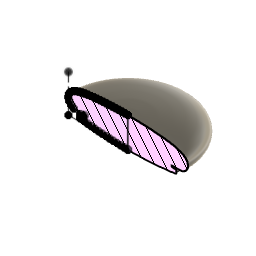
AirTag (Autodesk Fusion 360 design; units mm, degrees)
Autodesk Fusion 360 part; units mm, degrees
sketch "AirTag profile" plane through (0, 0, 0) normal (0, 1, 0) x (1, 0, 0)
  line L0 (-15.93, -10) -> (-15.93, 0) construction
  line L1 (0, 0) -> (-15.93, 0) construction
  line L2 (0, 0) -> (0, -7.98)
  line L3 (-12.72, -0.88) -> (-12.77, -0.93)
  line L4 (-12.77, -0.93) -> (-12.77, -1.84)
  line L5 (-12.77, -1.84) -> (-12.72, -1.89)
  line L6 (-12.72, -1.89) -> (-11.555, -1.89)
  line L7 (-11.555, -1.89) -> (-11.555, -2.29)
  line L8 (-11.555, -2.29) -> (-14.47, -2.29)
  spline S0 degree 5 poles (0, 0) (-0.0393, -0.0007) (-0.118, -0.002) (-0.2358, -0.0038) (-0.3929, -0.0059) (-0.589, -0.0078) (-0.7849, -0.0091) (-0.9807, -0.01) (-1.1764, -0.0108) (-1.3722, -0.0118) (-1.5682, -0.0134) (-1.7645, -0.0159) (-1.9612, -0.0197) (-2.1583, -0.0247) (-2.3557, -0.0307) (-2.5531, -0.0372) (-2.7505, -0.0438) (-2.9476, -0.05) (-3.1443, -0.0558) (-3.3406, -0.0612) (-3.5366, -0.0666) (-3.7323, -0.0726) (-3.928, -0.0796) (-4.1237, -0.0878) (-4.3195, -0.0972) (-4.5155, -0.1076) (-4.7117, -0.1186) (-4.9081, -0.1299) (-5.1045, -0.1412) (-5.3009, -0.1527) (-5.4971, -0.1645) (-5.6928, -0.1768) (-5.8881, -0.1897) (-6.083, -0.2033) (-6.2776, -0.2175) (-6.4721, -0.2319) (-6.6668, -0.2462) (-6.8618, -0.2602) (-7.0572, -0.2738) (-7.2531, -0.2872) (-7.4492, -0.3007) (-7.6454, -0.3148) (-7.8415, -0.3298) (-8.0375, -0.346) (-8.2332, -0.3634) (-8.4289, -0.3817) (-8.6245, -0.4006) (-8.8204, -0.42) (-9.0164, -0.4395) (-9.2124, -0.4592) (-9.4083, -0.4791) (-9.6039, -0.4992) (-9.799, -0.5198) (-9.9937, -0.5408) (-10.188, -0.5624) (-10.3822, -0.5846) (-10.5765, -0.6071) (-10.7711, -0.6301) (-10.9661, -0.6533) (-11.1616, -0.6769) (-11.3573, -0.7008) (-11.5532, -0.7251) (-11.7489, -0.7497) (-11.9442, -0.7748) (-12.139, -0.8004) (-12.3333, -0.8264) (-12.4883, -0.8476) (-12.6043, -0.8637) (-12.6814, -0.8746) (-12.72, -0.88) knots 0 0 0 0 0 0 0.01538462 0.03076923 0.04615385 0.06153846 0.07692308 0.09230769 0.10769231 0.12307692 0.13846154 0.15384615 0.16923077 0.18461538 0.2 0.21538462 0.23076923 0.24615385 0.26153846 0.27692308 0.29230769 0.30769231 0.32307692 0.33846154 0.35384615 0.36923077 0.38461538 0.4 0.41538462 0.43076923 0.44615385 0.46153846 0.47692308 0.49230769 0.50769231 0.52307692 0.53846154 0.55384615 0.56923077 0.58461538 0.6 0.61538462 0.63076923 0.64615385 0.66153846 0.67692308 0.69230769 0.70769231 0.72307692 0.73846154 0.75384615 0.76923077 0.78461538 0.8 0.81538462 0.83076923 0.84615385 0.86153846 0.87692308 0.89230769 0.90769231 0.92307692 0.93846154 0.95384615 0.96923077 0.98461538 1 1 1 1 1 1
  spline S1 degree 5 poles (-14.47, -2.29) (-14.4999, -2.3052) (-14.5592, -2.3362) (-14.6468, -2.3846) (-14.7609, -2.4529) (-14.8991, -2.5447) (-15.0325, -2.643) (-15.1609, -2.7478) (-15.2835, -2.8595) (-15.3993, -2.9782) (-15.5072, -3.1043) (-15.6057, -3.238) (-15.6936, -3.3793) (-15.7695, -3.5277) (-15.8323, -3.6825) (-15.8811, -3.8424) (-15.9152, -4.0061) (-15.934, -4.172) (-15.9374, -4.3386) (-15.9254, -4.5046) (-15.8984, -4.6687) (-15.8567, -4.8296) (-15.8012, -4.9864) (-15.7327, -5.138) (-15.6519, -5.2835) (-15.56, -5.4222) (-15.458, -5.5536) (-15.347, -5.6772) (-15.2281, -5.793) (-15.1023, -5.9012) (-14.9707, -6.0023) (-14.8344, -6.0968) (-14.6941, -6.1854) (-14.5505, -6.2687) (-14.4043, -6.3469) (-14.2558, -6.4204) (-14.1053, -6.4894) (-13.953, -6.5541) (-13.7991, -6.6147) (-13.6439, -6.6715) (-13.4874, -6.7249) (-13.3299, -6.7754) (-13.1715, -6.8231) (-13.0124, -6.8686) (-12.8527, -6.9121) (-12.6925, -6.9538) (-12.5319, -6.9939) (-12.3711, -7.0325) (-12.2099, -7.0696) (-12.0483, -7.1053) (-11.8864, -7.1393) (-11.7239, -7.1716) (-11.561, -7.2021) (-11.3975, -7.2308) (-11.2337, -7.2579) (-11.0698, -7.2835) (-10.9058, -7.3079) (-10.7419, -7.3313) (-10.5782, -7.354) (-10.4145, -7.3762) (-10.2507, -7.3981) (-10.0865, -7.4197) (-9.9219, -7.4411) (-9.7567, -7.4623) (-9.5913, -7.483) (-9.4257, -7.5031) (-9.2603, -7.5224) (-9.0954, -7.5407) (-8.9309, -7.5581) (-8.7668, -7.5745) (-8.6028, -7.5903) (-8.4386, -7.6056) (-8.2739, -7.6206) (-8.1087, -7.6354) (-7.9431, -7.6499) (-7.7772, -7.664) (-7.6115, -7.6776) (-7.446, -7.6905) (-7.2811, -7.7027) (-7.1166, -7.7145) (-6.9524, -7.7262) (-6.7882, -7.7381) (-6.6238, -7.7504) (-6.459, -7.7631) (-6.2937, -7.7759) (-6.128, -7.7884) (-5.9619, -7.8001) (-5.7957, -7.8106) (-5.6295, -7.8198) (-5.4634, -7.8278) (-5.2976, -7.8353) (-5.1321, -7.8425) (-4.9671, -7.85) (-4.8025, -7.858) (-4.638, -7.8664) (-4.4737, -7.8749) (-4.3091, -7.883) (-4.1443, -7.8905) (-3.979, -7.897) (-3.8134, -7.903) (-3.6475, -7.9085) (-3.4815, -7.9141) (-3.3154, -7.9201) (-3.1495, -7.9265) (-2.9837, -7.9332) (-2.818, -7.9397) (-2.6524, -7.9456) (-2.4868, -7.9504) (-2.3211, -7.954) (-2.1553, -7.9563) (-1.9895, -7.9579) (-1.8237, -7.9589) (-1.6578, -7.9599) (-1.492, -7.9613) (-1.3262, -7.963) (-1.1604, -7.9651) (-0.9947, -7.9675) (-0.8289, -7.97) (-0.6632, -7.9725) (-0.4974, -7.9748) (-0.3316, -7.9768) (-0.199, -7.9782) (-0.0995, -7.9792) (-0.0332, -7.9797) (0, -7.98) knots 0 0 0 0 0 0 0.00833333 0.01666667 0.025 0.03333333 0.04166667 0.05 0.05833333 0.06666667 0.075 0.08333333 0.09166667 0.1 0.10833333 0.11666667 0.125 0.13333333 0.14166667 0.15 0.15833333 0.16666667 0.175 0.18333333 0.19166667 0.2 0.20833333 0.21666667 0.225 0.23333333 0.24166667 0.25 0.25833333 0.26666667 0.275 0.28333333 0.29166667 0.3 0.30833333 0.31666667 0.325 0.33333333 0.34166667 0.35 0.35833333 0.36666667 0.375 0.38333333 0.39166667 0.4 0.40833333 0.41666667 0.425 0.43333333 0.44166667 0.45 0.45833333 0.46666667 0.475 0.48333333 0.49166667 0.5 0.50833333 0.51666667 0.525 0.53333333 0.54166667 0.55 0.55833333 0.56666667 0.575 0.58333333 0.59166667 0.6 0.60833333 0.61666667 0.625 0.63333333 0.64166667 0.65 0.65833333 0.66666667 0.675 0.68333333 0.69166667 0.7 0.70833333 0.71666667 0.725 0.73333333 0.74166667 0.75 0.75833333 0.76666667 0.775 0.78333333 0.79166667 0.8 0.80833333 0.81666667 0.825 0.83333333 0.84166667 0.85 0.85833333 0.86666667 0.875 0.88333333 0.89166667 0.9 0.90833333 0.91666667 0.925 0.93333333 0.94166667 0.95 0.95833333 0.96666667 0.975 0.98333333 0.99166667 1 1 1 1 1 1
  point P0 (-15.93, 0)
  point P1 (0, -7.98)
  point P2 (-0.83, -7.97)
  point P3 (-1.66, -7.96)
  point P4 (-3.32, -7.92)
  point P5 (-2.49, -7.95)
  point P6 (-4.15, -7.89)
  point P7 (-7.45, -7.69)
  point P8 (-6.63, -7.75)
  point P9 (-4.97, -7.85)
  point P10 (-5.8, -7.81)
  point P11 (-8.28, -7.62)
  point P12 (-9.1, -7.54)
  point P13 (-9.93, -7.44)
  point P14 (-10.75, -7.33)
  point P15 (-11.57, -7.2)
  point P16 (-12.38, -7.03)
  point P17 (-13.96, -6.55)
  point P18 (-14.7, -6.18)
  point P19 (-15.8, -4.98)
  point P20 (-15.93, -4.17)
  point P21 (-12.72, -0.88)
  point P22 (-13.18, -6.82)
  point P23 (-15.35, -5.67)
  point P24 (-14.47, -2.29)
  point P25 (-15.16, -2.75)
  point P26 (-15.69, -3.38)
  point P27 (-11.75, -0.75)
  point P28 (-10.77, -0.63)
  point P29 (-9.8, -0.52)
  point P30 (-8.82, -0.42)
  point P31 (-7.84, -0.33)
  point P32 (-6.86, -0.26)
  point P33 (-5.89, -0.19)
  point P34 (-4.91, -0.13)
  point P35 (-3.93, -0.08)
  point P36 (-2.95, -0.05)
  point P37 (-0.98, -0.01)
  point P38 (-1.96, -0.02)
  point P39 (-11.555, -2.29)
  point P40 (-11.555, -1.89)
  point P41 (-12.77, -1.84)
  point P42 (-12.72, -1.89)
  point P43 (-12.77, -0.93)
  point P44 (-0.98, -0.01)
  point P45 (-1.96, -0.02)
  point P46 (-2.95, -0.05)
  point P47 (-3.93, -0.08)
  point P48 (-4.91, -0.13)
  point P49 (-5.89, -0.19)
  point P50 (-6.86, -0.26)
  point P51 (-7.84, -0.33)
  point P52 (-8.82, -0.42)
  point P53 (-9.8, -0.52)
  point P54 (-10.77, -0.63)
  point P55 (-11.75, -0.75)
  point P56 (-15.16, -2.75)
  point P57 (-15.69, -3.38)
  point P58 (-15.93, -4.17)
  point P59 (-15.8, -4.98)
  point P60 (-15.35, -5.67)
  point P61 (-14.7, -6.18)
  point P62 (-13.96, -6.55)
  point P63 (-13.18, -6.82)
  point P64 (-12.38, -7.03)
  point P65 (-11.57, -7.2)
  point P66 (-10.75, -7.33)
  point P67 (-9.93, -7.44)
  point P68 (-9.1, -7.54)
  point P69 (-8.28, -7.62)
  point P70 (-7.45, -7.69)
  point P71 (-6.63, -7.75)
  point P72 (-5.8, -7.81)
  point P73 (-4.97, -7.85)
  point P74 (-4.15, -7.89)
  point P75 (-3.32, -7.92)
  point P76 (-2.49, -7.95)
  point P77 (-1.66, -7.96)
  point P78 (-0.83, -7.97)
  dimension "d1" = 10
  dimension "d2" = 15.93
  dimension "d3" = 15.93
  dimension "d4" = 15.1
  dimension "d5" = 14.27
  dimension "d6" = 13.44
  dimension "d7" = 12.61
  dimension "d8" = 11.78
  dimension "d9" = 10.96
  dimension "d10" = 10.13
  dimension "d11" = 9.3
  dimension "d12" = 8.48
  dimension "d13" = 7.65
  dimension "d14" = 6.83
  dimension "d15" = 6
  dimension "d16" = 5.18
  dimension "d17" = 4.36
  dimension "d18" = 3.55
  dimension "d19" = 2.75
  dimension "d20" = 1.97
  dimension "d21" = 1.23
  dimension "d22" = 0.58
  dimension "d23" = 0.13
  dimension "d24" = 7.98
  dimension "d25" = 7.97
  dimension "d26" = 7.96
  dimension "d27" = 7.95
  dimension "d28" = 7.92
  dimension "d29" = 7.89
  dimension "d30" = 7.85
  dimension "d31" = 7.81
  dimension "d32" = 7.75
  dimension "d33" = 7.69
  dimension "d34" = 7.62
  dimension "d35" = 7.54
  dimension "d36" = 7.44
  dimension "d37" = 7.33
  dimension "d38" = 7.2
  dimension "d39" = 7.03
  dimension "d40" = 6.82
  dimension "d41" = 6.55
  dimension "d42" = 6.18
  dimension "d43" = 5.67
  dimension "d44" = 4.98
  dimension "d45" = 4.17
  dimension "d46" = 0.24
  dimension "d47" = 0.77
  dimension "d48" = 1.46
  dimension "d49" = 3.21
  dimension "d50" = 4.18
  dimension "d51" = 5.16
  dimension "d52" = 6.13
  dimension "d53" = 7.11
  dimension "d54" = 8.09
  dimension "d55" = 9.07
  dimension "d56" = 10.04
  dimension "d57" = 11.02
  dimension "d58" = 12
  dimension "d59" = 12.98
  dimension "d60" = 13.97
  dimension "d61" = 14.95
  dimension "d62" = 15.93
  dimension "d63" = 0.01
  dimension "d64" = 0.02
  dimension "d65" = 0.05
  dimension "d66" = 0.08
  dimension "d67" = 0.13
  dimension "d68" = 0.19
  dimension "d69" = 0.26
  dimension "d70" = 0.33
  dimension "d71" = 0.42
  dimension "d72" = 0.52
  dimension "d73" = 0.63
  dimension "d74" = 0.75
  dimension "d75" = 0.88
  dimension "d76" = 2.29
  dimension "d77" = 2.75
  dimension "d78" = 3.38
  dimension "d79" = 11.555
  dimension "d80" = 2.29
  dimension "d81" = 1.89
  dimension "d82" = 0.05
  dimension "d83" = 0.05
  dimension "d84" = 0.05
  constraint vertical L0
  constraint horizontal L1.start L0.end
  constraint coincident L1.start L2.start
  constraint coincident P0 L0.end
  constraint coincident L0 P58
  constraint coincident P1 L2.end
  constraint vertical P39 P40
  constraint vertical P21 P42
  constraint horizontal P40 P42
  constraint vertical P41 P43
  constraint coincident P21 L3.start
  constraint coincident P43 L3.end
  constraint coincident P41 L4.end
  constraint coincident P42 L5.end
  constraint coincident P40 L6.end
  constraint coincident P39 L7.end
  constraint coincident P24 L8.end
  constraint coincident P44 P37
  constraint coincident P45 P38
  constraint coincident P46 P36
  constraint coincident P47 P35
  constraint coincident P48 P34
  constraint coincident P49 P33
  constraint coincident P50 P32
  constraint coincident P51 P31
  constraint coincident P52 P30
  constraint coincident P53 P29
  constraint coincident P54 P28
  constraint coincident P55 P27
  constraint coincident P56 P25
  constraint coincident P57 P26
  constraint coincident P58 P20
  constraint coincident P59 P19
  constraint coincident P60 P23
  constraint coincident P61 P18
  constraint coincident P62 P17
  constraint coincident P63 P22
  constraint coincident P64 P16
  constraint coincident P65 P15
  constraint coincident P66 P14
  constraint coincident P67 P13
  constraint coincident P68 P12
  constraint coincident P69 P11
  constraint coincident P70 P7
  constraint coincident P71 P8
  constraint coincident P72 P10
  constraint coincident P73 P9
  constraint coincident P74 P6
  constraint coincident P75 P4
  constraint coincident P76 P5
  constraint coincident P77 P3
  constraint coincident P78 P2
  constraint coincident P0 L1
  measures "d1" distance of L0.start P0
  measures "d2" distance of L1.start L0
  measures "d3" distance of L0 P1
  measures "d4" distance of L0 P78
  measures "d5" distance of L0 P77
  measures "d6" distance of L0 P76
  measures "d7" distance of L0 P75
  measures "d8" distance of L0 P74
  measures "d9" distance of L0 P73
  measures "d10" distance of L0 P72
  measures "d11" distance of L0 P71
  measures "d12" distance of L0 P70
  measures "d13" distance of L0 P69
  measures "d14" distance of L0 P68
  measures "d15" distance of L0 P67
  measures "d16" distance of L0 P66
  measures "d17" distance of L0 P65
  measures "d18" distance of L0 P64
  measures "d19" distance of L0 P63
  measures "d20" distance of L0 P62
  measures "d21" distance of L0 P61
  measures "d22" distance of L0 P60
  measures "d23" distance of L0 P59
  measures "d24" distance of L1.start P1
  measures "d25" distance of P78 L1
  measures "d26" distance of P77 L1
  measures "d27" distance of P76 L1
  measures "d28" distance of P75 L1
  measures "d29" distance of P74 L1
  measures "d30" distance of P73 L1
  measures "d31" distance of P72 L1
  measures "d32" distance of P71 L1
  measures "d33" distance of P70 L1
  measures "d34" distance of P69 L1
  measures "d35" distance of P68 L1
  measures "d36" distance of P67 L1
  measures "d37" distance of P66 L1
  measures "d38" distance of P65 L1
  measures "d39" distance of P64 L1
  measures "d40" distance of P63 L1
  measures "d41" distance of P62 L1
  measures "d42" distance of P61 L1
  measures "d43" distance of P60 L1
  measures "d44" distance of P59 L1
  measures "d45" distance of P58 L1
  measures "d46" distance of L0 P57
  measures "d47" distance of L0 P56
  measures "d48" distance of L0 P24
  measures "d49" distance of L0 P21
  measures "d50" distance of L0 P55
  measures "d51" distance of L0 P54
  measures "d52" distance of L0 P53
  measures "d53" distance of L0 P52
  measures "d54" distance of L0 P51
  measures "d55" distance of L0 P50
  measures "d56" distance of L0 P49
  measures "d57" distance of L0 P48
  measures "d58" distance of L0 P47
  measures "d59" distance of L0 P46
  measures "d60" distance of L0 P45
  measures "d61" distance of L0 P44
  measures "d62" distance of L0 L1.start
  measures "d63" distance of L1 P44
  measures "d64" distance of L1 P45
  measures "d65" distance of L1 P46
  measures "d66" distance of L1 P47
  measures "d67" distance of L1 P48
  measures "d68" distance of L1 P49
  measures "d69" distance of L1 P50
  measures "d70" distance of L1 P51
  measures "d71" distance of L1 P52
  measures "d72" distance of L1 P53
  measures "d73" distance of P54 L1
  measures "d74" distance of P55 L1
  measures "d75" distance of P21 L1
  measures "d76" distance of P24 L1
  measures "d77" distance of P56 L1
  measures "d78" distance of P57 L1
  measures "d79" distance of L2 P39
  measures "d80" distance of L1 P39
  measures "d81" distance of L1 P40
  measures "d82" horizontal distance of P41 P42
  measures "d83" vertical distance of P41 P42
  measures "d84" vertical distance of P21 P43
revolve "Revolve1" add sketch "AirTag profile" angle 360 about axis through (0, 0, 0) along (0, 0, 1)
equation "d3 = d2"
equation "d79 = ( 23.11 / 2 ) * 1 mm"
named bodies: "AirTag"
